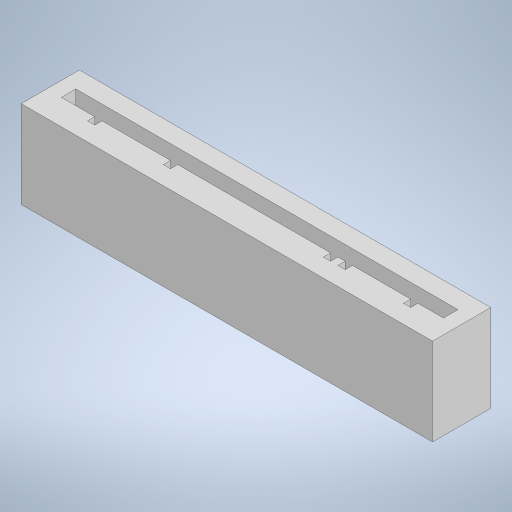
# Autodesk Inventor part: Better Breakout
Saved by Autodesk Inventor 2024.1 (Build 281209000, 209)
## iProperties
Created: 2024-01-16
Part Number: Better Breakout
Material: Generic
Document SubType Name: Modeling
Designer: ryanm
Density: 1 g/cm^3
Appearance: Default
Author: ryanm
Autodesk Inventor part; units mm, degrees
ref_plane "YZ Plane" through (0, 0, 0) normal (1, 0, 0) x (0, 1, 0)
ref_plane "XZ Plane" through (0, 0, 0) normal (0, 1, 0) x (-1, 0, 0)
ref_plane "XY Plane" through (0, 0, 0) normal (0, 0, 1) x (1, 0, 0)
sketch "Sketch1" plane through (0, 0, 0) normal (0, 1, 0) x (-1, 0, 0)
  line L0 (28.25, -4) -> (-28.25, -4)
  line L1 (-28.25, -4) -> (-28.25, 4)
  line L2 (-28.25, 4) -> (28.25, 4)
  line L3 (28.25, 4) -> (28.25, -4)
  point P0 (0, 0)
  point P1 (0, -4)
  point P2 (28.25, 0)
  dimension "d1" = 56.5
  dimension "d2" = 8
  constraints: 8 end point, 2 midpoint, 2 parallel, 1 horizontal, 1 horizontal alignment, 1 perpendicular, 1 vertical alignment
  measures "d1" distance of L0.start L0.end
  measures "d2" distance of L2.end L0.start
extrude "Extrusion1" add sketch "Sketch1" along normal blind 12
sketch "Sketch2" plane through (0, 12, 0) normal (0, 1, 0) x (1, 0, 0)
  line L0 (-26.25, 1.5) -> (26.25, 1.5)
  line L1 (26.25, 1.5) -> (26.25, -0.5)
  line L2 (26.25, -0.5) -> (-26.25, -0.5)
  line L3 (-26.25, -0.5) -> (-26.25, 1.5)
  line L4 (28.25, 4) -> (-28.25, 4) projected
  line L5 (28.25, -4) -> (28.25, 4) projected
  point P0 (0, 0)
  point P1 (0, 1.5)
  dimension "d5" = 2.5
  dimension "d6" = 2
  dimension "d7" = 2
  constraints: 8 end point, 2 parallel, 1 horizontal, 1 midpoint, 1 perpendicular, 1 vertical alignment
  measures "d5" distance between parallel lines of L0 L4
  measures "d6" distance of L2.end L0.start
  measures "d7" distance between parallel lines of L5 L1
extrude "Extrusion2" cut sketch "Sketch2" against normal blind 8.6
sketch "Sketch3" plane through (0, 3.4, 0) normal (0, 1, 0) x (1, 0, 0)
  line L0 (26.25, -0.5) -> (-26.25, -0.5) projected
  line L1 (26.25, 1.5) -> (26.25, -0.5) projected
  line L2 (-26.25, 1.5) -> (26.25, 1.5) projected
  line L3 (-26.25, -0.5) -> (-26.25, 1.5) projected
  line L4 (-25.25, 1.5) -> (-25.25, -0.5)
  line L5 (25.25, 1.5) -> (25.25, -0.5)
  point P0 (0, 0)
  dimension "d10" = 1
  dimension "d11" = 1
  constraints: 4 end point, 4 point on line, 1 perpendicular, 1 vertical
  measures "d10" distance between parallel lines of L4 L3
  measures "d11" distance between parallel lines of L1 L5
extrude "Extrusion3" cut sketch "Sketch3" against normal through all contours L0 L4 L2 L5
sketch "Sketch5" plane through (26.25, 12, 0.5) normal (0, 0, -1) x (-1, 0, 0)
  line L0 (52.5, 0) -> (0, 0) projected
  line L1 (52.5, 0) -> (52.5, -8.6) projected
  line L2 (52.5, -8.6) -> (51.5, -8.6) projected
  line L3 (51.5, -8.6) -> (51.5, -12) projected
  line L4 (1, -12) -> (51.5, -12) projected
  line L5 (1, -8.6) -> (1, -12) projected
  line L6 (1, -8.6) -> (0, -8.6) projected
  line L7 (0, 0) -> (0, -8.6) projected
  line L8 (51.5, -8.6) -> (1, -8.6)
  point P0 (26.25, -12)
  constraints: 2 end point, 1 horizontal
extrude "Extrusion4" cut sketch "Sketch5" along normal through all both and the other way through all contours L3 L4 L5 L8
sketch "Sketch6" plane through (-25.25, 3.4, 0.5) normal (0, -1, 0) x (1, 0, 0)
  line L0 (0, 3.5) -> (50.5, 3.5) projected
  line L1 (0, 3.5) -> (0, 0) projected
  line L2 (50.5, 0) -> (0, 0) projected
  line L3 (50.5, 3.5) -> (50.5, 0) projected
  line L4 (3.6, 0) -> (3.6, 1)
  line L5 (3.6, 1) -> (4.6, 1)
  line L6 (4.6, 1) -> (4.6, 0)
  line L7 (14, 0) -> (14, 1)
  line L8 (14, 1) -> (15, 1)
  line L9 (15, 1) -> (15, 0)
  line L10 (36, 0) -> (36, 1)
  line L11 (36, 1) -> (37, 1)
  line L12 (37, 1) -> (37, 0)
  line L13 (38, 0) -> (38, 1)
  line L14 (38, 1) -> (39, 1)
  line L15 (39, 1) -> (39, 0)
  line L16 (47, 0) -> (47, 1)
  line L17 (47, 1) -> (48, 1)
  line L18 (48, 1) -> (48, 0)
  point P0 (25.25, -0.5)
  dimension "d16" = 1
  dimension "d17" = 3.6
  dimension "d18" = 14
  dimension "d19" = 36
  dimension "d20" = 38
  dimension "d21" = 47
  constraints: 30 end point, 8 vertical, 7 equal length, 4 point on line, 3 perpendicular, 2 parallel, 11 other
  measures "d16" distance of L4.start L4.end
  measures "d17" distance between parallel lines of L1 L4
  measures "d18" distance between parallel lines of L1 L7
  measures "d19" distance between parallel lines of L1 L10
  measures "d20" distance between parallel lines of L1 L13
  measures "d21" distance between parallel lines of L1 L16
extrude "Extrusion5" cut sketch "Sketch6" against normal up to surface (8.6 mm away) contours L4 L5 L6 L2 | L2 L16 L17 L18 | L7 L8 L9 L2 | L2 L13 L14 L15 | L10 L11 L12 L2
sketch "Sketch7" plane through (-25.25, 3.4, 4) normal (0, -1, 0) x (1, 0, 0)
  line L0 (36, -3.5) -> (36, -2.5) projected
  line L1 (36, -2.5) -> (37, -2.5) projected
  line L2 (37, -2.5) -> (37, -3.5) projected
  line L3 (38, -3.5) -> (37, -3.5) projected
  line L4 (38, -3.5) -> (38, -2.5) projected
  line L5 (38, -2.5) -> (39, -2.5) projected
  line L6 (39, -2.5) -> (39, -3.5) projected
  line L7 (47, -3.5) -> (39, -3.5) projected
  line L8 (47, -3.5) -> (47, -2.5) projected
  line L9 (47, -2.5) -> (48, -2.5) projected
  line L10 (48, -2.5) -> (48, -3.5) projected
  line L11 (50.5, -3.5) -> (48, -3.5) projected
  line L12 (50.5, 0) -> (50.5, -3.5) projected
  line L13 (0, 0) -> (50.5, 0) projected
  line L14 (0, 0) -> (0, -3.5) projected
  line L15 (3.6, -3.5) -> (0, -3.5) projected
  line L16 (3.6, -3.5) -> (3.6, -2.5) projected
  line L17 (3.6, -2.5) -> (4.6, -2.5) projected
  line L18 (4.6, -2.5) -> (4.6, -3.5) projected
  line L19 (14, -3.5) -> (4.6, -3.5) projected
  line L20 (14, -3.5) -> (14, -2.5) projected
  line L21 (14, -2.5) -> (15, -2.5) projected
  line L22 (15, -2.5) -> (15, -3.5) projected
  line L23 (36, -3.5) -> (15, -3.5) projected
  point P0 (25.25, -4)
extrude "Extrusion6" add sketch "Sketch7" along normal up to surface (3.4 mm away)
sketch "Sketch8" plane through (26.25, 3.4, 0.5) normal (0, 0, -1) x (-1, 0, 0)
  line L0 (3.5, 8.6) -> (3.5, -3.4) projected
  line L1 (0, 8.6) -> (3.5, 8.6) projected
  line L2 (0, 8.6) -> (0, 0) projected
  line L3 (0, 0) -> (1, 0) projected
  line L4 (1, -3.4) -> (1, 0) projected
  line L5 (3.5, -3.4) -> (1, -3.4) projected
  line L6 (4.5, 8.6) -> (4.5, -3.4) projected
  line L7 (12.5, -3.4) -> (4.5, -3.4) projected
  line L8 (12.5, 8.6) -> (12.5, -3.4) projected
  line L9 (4.5, 8.6) -> (12.5, 8.6) projected
  line L10 (15.5, 8.6) -> (15.5, -3.4) projected
  line L11 (36.5, -3.4) -> (15.5, -3.4) projected
  line L12 (36.5, -3.4) -> (36.5, 8.6) projected
  line L13 (15.5, 8.6) -> (36.5, 8.6) projected
  line L14 (14.5, -3.4) -> (14.5, 8.6) projected
  line L15 (13.5, 8.6) -> (14.5, 8.6) projected
  line L16 (13.5, 8.6) -> (13.5, -3.4) projected
  line L17 (14.5, -3.4) -> (13.5, -3.4) projected
  line L18 (46.9, -3.4) -> (46.9, 8.6) projected
  line L19 (37.5, 8.6) -> (46.9, 8.6) projected
  line L20 (37.5, 8.6) -> (37.5, -3.4) projected
  line L21 (46.9, -3.4) -> (37.5, -3.4) projected
  line L22 (47.9, 8.6) -> (47.9, -3.4) projected
  line L23 (51.5, -3.4) -> (47.9, -3.4) projected
  line L24 (51.5, 0) -> (51.5, -3.4) projected
  line L25 (51.5, 0) -> (52.5, 0) projected
  line L26 (52.5, 8.6) -> (52.5, 0) projected
  line L27 (47.9, 8.6) -> (52.5, 8.6) projected
  line L28 (51.5, 0) -> (1, 0) projected
  line L29 (2.2, -3.4) -> (5.8, -3.4)
  line L30 (5.8, -3.4) -> (5.8, 0)
  line L31 (5.8, 0) -> (2.2, 0)
  line L32 (2.2, 0) -> (2.2, -3.4)
  line L33 (11.2, 0) -> (16.8, 0)
  line L34 (16.8, 0) -> (16.8, -3.4)
  line L35 (16.8, -3.4) -> (11.2, -3.4)
  line L36 (11.2, -3.4) -> (11.2, 0)
  line L37 (1, 0) -> (51.5, 0) projected
  line L38 (35.2, 0) -> (38.8, 0)
  line L39 (38.8, 0) -> (38.8, -3.4)
  line L40 (38.8, -3.4) -> (35.2, -3.4)
  line L41 (35.2, -3.4) -> (35.2, 0)
  line L42 (45.6, 0) -> (49.2, 0)
  line L43 (49.2, 0) -> (49.2, -3.4)
  line L44 (49.2, -3.4) -> (45.6, -3.4)
  line L45 (45.6, -3.4) -> (45.6, 0)
  point P0 (26.25, -3.4)
  point P1 (4, -3.4)
  point P2 (4, 0)
  point P3 (2.2, 0)
  point P4 (11.2, -3.4)
  dimension "d26" = 3.6
  dimension "d27" = 1.3
  dimension "d30" = 1.3
  dimension "d31" = 1.3
  dimension "d32" = 1.3
  dimension "d33" = 1.3
  dimension "d34" = 1.3
  dimension "d35" = 1.3
  constraints: 32 end point, 8 parallel, 6 point on line, 4 horizontal, 4 perpendicular, 2 midpoint, 1 vertical alignment, 3 other
  measures "d26" distance between parallel lines of L30 L32
  measures "d27" distance between parallel lines of L0 L32
  measures "d30" distance between parallel lines of L36 L8
  measures "d31" distance between parallel lines of L34 L10
  measures "d32" distance between parallel lines of L41 L12
  measures "d33" distance between parallel lines of L39 L20
  measures "d34" distance between parallel lines of L18 L45
  measures "d35" distance between parallel lines of L43 L22
extrude "Extrusion7" cut sketch "Sketch8" against normal blind 1.5 contours L28 L6 L29 L0 | L0 L5 L32 L28 | L28 L30 L7 L6 | L28 L8 L7 L36 | L28 L16 L35 L8 | L28 L14 L17 L16 | L28 L10 L35 L14 | L28 L34 L11 L10 | L28 L12 L11 L41 | L28 L20 L40 L12 | L28 L39 L21 L20 | L28 L18 L21 L45 | L28 L22 L44 L18 | L28 L43 L23 L22
equation "\"d11\" = d10"
equation "\"d33\" = d32"
equation "\"d34\" = d33"
equation "\"d35\" = d34"
body "Solid1"
